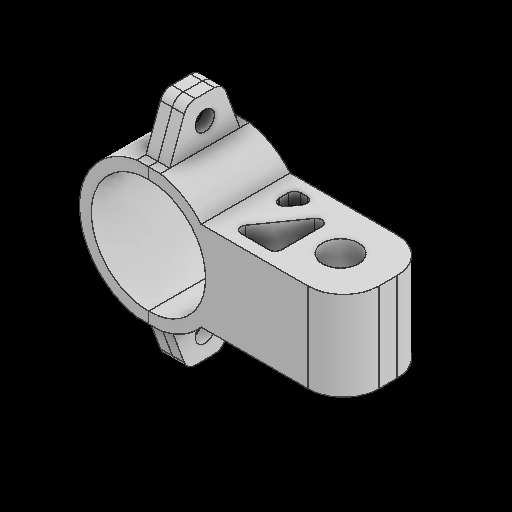
# Autodesk Inventor part: ScreenMount
Saved by Autodesk Inventor 2025.2 (Build 292293000, 293)
## iProperties
Created: 2026-06-24
Part Number: ScreenMount
Material: Generic
Document SubType Name: Modeling
Designer: valer
Density: 1 g/cm^3
Appearance: Default
Author: valer
Autodesk Inventor part; units mm, degrees
ref_plane "YZ Plane" through (0, 0, 0) normal (1, 0, 0) x (0, 1, 0)
ref_plane "XZ Plane" through (0, 0, 0) normal (0, 1, 0) x (-1, 0, 0)
ref_plane "XY Plane" through (0, 0, 0) normal (0, 0, 1) x (1, 0, 0)
sketch "Base" plane through (0, 0, 0) normal (0, 0, 1) x (1, 0, 0)
  circle A0 centre (0, 0) radius 9.625
  circle A1 centre (0, 0) radius 11.625
  line L0 (0, 11.625) -> (0, 19.4517)
  line L1 (0, 19.4517) -> (2, 19.4517)
  line L2 (2, 19.4517) -> (2, 11.4517)
  line L3 (0, -27.2323) -> (0, 27.2323) projected
  line L4 (-16.275, 0) -> (16.275, 0) construction
  line L5 (0, -11.625) -> (0, -19.4517)
  line L6 (0, -19.4517) -> (2, -19.4517)
  line L7 (2, -19.4517) -> (2, -11.4517)
  line L8 (0, 19.4517) -> (-2, 19.4517)
  line L9 (-2, 19.4517) -> (-2, 11.4517)
  line L10 (0, -19.4517) -> (-2, -19.4517)
  line L11 (-2, -19.4517) -> (-2, -11.4517)
  point P0 (0, 9.625)
  point P1 (0, -9.625)
  dimension "d0" = 19.25
  dimension "d1" = 2
  dimension "d2" = 2
  dimension "d3" = 8
  constraints: 20 end point, 8 symmetric about line, 2 centre point, 2 coincident, 2 perpendicular, 2 point on circle, 1 collinear, 1 vertical
  measures "d0" diameter of A0
  measures "d1" radial gap between concentric circles of A0 A1
  measures "d2" distance between parallel lines of L2 L0
  measures "d3" distance of L1.end L2.end
extrude "BaseFeature" add sketch "Base" along normal blind 15 contours A0 L3 A1 | L0 L1 L2 A1 | A1 L7 L6 L3 picked at (10.7732, -1.6086)
extrude "HalfFeature" add sketch "Base" along normal blind 15 separate body contours A0 L3 A1 | A1 L9 L8 L0 | L3 L10 L11 A1 picked at (-2.9644, 10.4925)
sketch "Ears" plane through (2, 11.4517, 0) normal (1, 0, 0) x (0, 0, -1)
  line L0 (0, 0) -> (0, 8) projected
  line L1 (0, 8) -> (-15, 8) projected
  line L2 (-15, 0) -> (-15, 8) projected
  line L3 (0, 0) -> (-15, 0) projected
  line L4 (0, -30.9033) -> (0, -22.9033) projected
  line L5 (0, -22.9033) -> (-15, -22.9033) projected
  line L6 (-15, -30.9033) -> (-15, -22.9033) projected
  line L7 (0, -30.9033) -> (-15, -30.9033) projected
  line L8 (-13.4118, 0) -> (-10.5, 8)
  line L9 (-7.5, -30.9033) -> (-7.5, 8) construction
  line L10 (-15, -21.0767) -> (-15, -1.8267) projected
  line L11 (-15, -11.4517) -> (0, -11.4517) construction
  line L12 (0, -21.0767) -> (0, -1.8267) projected
  line L13 (-13.4118, -22.9033) -> (-10.5, -30.9033)
  line L14 (-1.5882, 0) -> (-4.5, 8)
  line L15 (-1.5882, -22.9033) -> (-4.5, -30.9033)
  dimension "d8" = 70
  dimension "d9" = 6
  constraints: 12 end point, 6 symmetric about line, 3 midpoint, 2 point on line, 1 perpendicular
  measures "d8" angle of L1 L8
  measures "d9" distance of L14.end L8.end
extrude "BaseEarsFeature" cut sketch "Ears" against normal through all contours L3 L14 L1 L0 | L3 L2 L1 L8 | L7 L15 L5 L4 | L7 L6 L5 L13 bodies 1
extrude "HalfEarsFeatrue" cut sketch "Ears" against normal through all contours L3 L14 L1 L0 | L3 L2 L1 L8 | L7 L15 L5 L4 | L7 L6 L5 L13 bodies 2
fillet "EarFilletsFeature" radius 2 8 edges at (1, 19.4517, 10.5) (1, 19.4517, 4.5) (1, -19.4517, 10.5) (1, -19.4517, 4.5) (-1, 19.4517, 10.5) (-1, 19.4517, 4.5) (-1, -19.4517, 10.5) (-1, -19.4517, 4.5)
sketch "EarMountHoles" plane through (2, 11.4517, 13.4118) normal (1, 0, 0) x (0, 0, -1)
  arc A0 (9.3907, 6.684) -> (7.5113, 8) centre (7.5113, 6) ccw projected
  line L0 (7.5113, 8) -> (4.3122, 8) projected
  arc A1 (4.3122, 8) -> (2.4328, 6.684) centre (4.3122, 6) ccw projected
  line L1 (2.4328, 6.684) -> (0, 0) projected
  line L2 (11.8235, 0) -> (0, 0) projected
  line L3 (11.8235, 0) -> (9.3907, 6.684) projected
  circle A2 centre (5.9118, 4) radius 1.625
  line L4 (7.5113, -30.9033) -> (4.3122, -30.9033) projected
  line L5 (5.9118, -30.9033) -> (5.9118, 8) construction
  line L6 (-1.5882, -21.0767) -> (-1.5882, -1.8267) projected
  line L7 (-1.5882, -11.4517) -> (13.4118, -11.4517) construction
  circle A3 centre (5.9118, -26.9033) radius 1.625
  dimension "d15" = 3.25
  dimension "d16" = 4
  constraints: 4 end point, 3 midpoint, 2 centre point, 1 horizontal, 1 point on line, 1 symmetric about line, 1 other
  measures "d15" diameter of A2
  measures "d16" vertical distance of L0.end A2.centre
extrude "EarMountHolesHalfFeature" cut sketch "EarMountHoles" against normal through all contours A2 | A3 bodies 1
extrude "EarMountHolesOtherHalfFeature" cut sketch "EarMountHoles" against normal blind 10 contours A2 | A3 bodies 2
sketch "MonitorArmMount" plane through (0, 0, 15) normal (0, 0, 1) x (1, 0, 0)
  line L0 (-6.5764, 0) -> (39.4584, 0) projected
  line L1 (0, -27.2323) -> (0, 27.2323) projected
  arc A0 (2, -11.4517) -> (2, 11.4517) centre (0, 0) ccw projected
  line L2 (8.882, -7.5) -> (32.882, -7.5)
  line L3 (32.882, -7.5) -> (32.882, 7.5)
  line L4 (32.882, 7.5) -> (8.882, 7.5)
  point P0 (32.882, 0)
  dimension "d21" = 24
  dimension "d22" = 15
  constraints: 6 end point, 2 point on circle, 1 horizontal, 1 midpoint, 1 parallel, 1 perpendicular, 1 point on line
  measures "d21" distance of L2.start L2.end
  measures "d22" distance of L2.end L3.end
extrude "MonitorArmMountFeature" add sketch "MonitorArmMount" against normal up to surface (15 mm away) bodies 1
fillet "OutsideFilletsFeature" radius 6 2 edges at (32.882, 0, 15) (32.882, 0, 0)
sketch "MonitorMount" plane through (8.882, 7.5, 15) normal (0, 1, 0) x (1, 0, 0)
  arc A0 (24, 9) -> (18, 15) centre (18, 9) ccw projected
  line L0 (0, 15) -> (18, 15) projected
  line L1 (0, 0) -> (0, 15) projected
  line L2 (18, 0) -> (0, 0) projected
  arc A1 (18, 0) -> (24, 6) centre (18, 6) ccw projected
  line L3 (24, 6) -> (24, 9) projected
  circle A2 centre (16, 7.5) radius 3.05
  line L4 (24, 7.5) -> (0, 7.5) construction
  line L5 (0, 0) -> (0, 15) projected
  line L6 (24, 6) -> (24, 9) projected
  point P0 (-8.882, 15)
  dimension "d26" = 6.1
  dimension "d29" = 8
  constraints: 3 midpoint, 2 end point, 1 centre point, 1 perpendicular, 1 point on line
  measures "d26" diameter of A2
  measures "d29" distance of point (24, 7.5) A2.centre
extrude "MonitorMountFeature" cut sketch "MonitorMount" against normal through all contours A2 bodies 1
sketch "MountHoles" plane through (8.882, 7.5, 15) normal (0, 1, 0) x (1, 0, 0)
  circle A0 centre (16, 7.5) radius 3.05 projected
  arc A1 (24, 9) -> (18, 15) centre (18, 9) ccw projected
  line L0 (0, 15) -> (18, 15) projected
  line L1 (0, 0) -> (0, 15) projected
  line L2 (18, 0) -> (0, 0) projected
  arc A2 (18, 0) -> (24, 6) centre (18, 6) ccw projected
  line L3 (24, 6) -> (24, 9) projected
  line L4 (10.5, 13) -> (2.743, 2)
  line L5 (2.743, 2) -> (10.5, 2)
  line L6 (0.743, 0) -> (0.743, 15) projected
  line L7 (10.5, 2) -> (10.5, 13)
  line L8 (6.8291, 13) -> (2.743, 7.2056)
  line L9 (2.743, 7.2056) -> (2.743, 13)
  line L10 (2.743, 13) -> (6.8291, 13)
  line L11 (18, 0) -> (0, 0) projected
  line L12 (0, 15) -> (18, 15) projected
  line L13 (24, 6) -> (24, 9) projected
  line L14 (10.5, 13) -> (6.8291, 13)
  line L15 (2.743, 2) -> (2.743, 7.2056)
  point P0 (-8.882, 15)
  dimension "d30" = 3
  dimension "d31" = 2
  dimension "d32" = 2
  dimension "d33" = 2
  dimension "d34" = 5.5
  constraints: 16 end point, 5 parallel, 3 perpendicular, 2 collinear
  measures "d30" distance between parallel lines of L8 L4
  measures "d31" distance between parallel lines of L2 L5
  measures "d32" distance between parallel lines of L0 L10
  measures "d33" distance between parallel lines of L6 L15
  measures "d34" distance from line of A0.centre L7
extrude "MountHolesFeature" cut sketch "MountHoles" against normal through all contours L7 L5 L4 | L8 L9 L10 bodies 1
fillet "InsideFilletsFeature" radius 1 6 edges at (19.382, 0, 13) (11.625, 0, 13) (19.382, 0, 2) (15.7111, 0, 2) (11.625, 0, 7.7944) (11.625, 0, 2)
equation "\"d32\" = d31"
equation "\"d33\" = d31"
